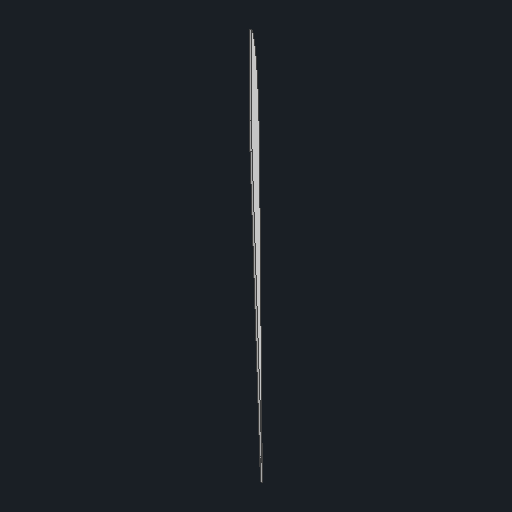
# Autodesk Inventor part: standoff
Saved by Autodesk Inventor 2023 (Build 270158030, 158C)
## iProperties
Created: 2022-03-24
Part Number: standoff
Material: Generic
Document SubType Name: Modeling
Designer: kardo
Density: 1 g/cm^3
Appearance: Default
Author: kardo
Autodesk Inventor part; units mm, degrees
ref_plane "YZ Plane" through (0, 0, 0) normal (1, 0, 0) x (0, 1, 0)
ref_plane "XZ Plane" through (0, 0, 0) normal (0, 1, 0) x (-1, 0, 0)
ref_plane "XY Plane" through (0, 0, 0) normal (0, 0, 1) x (1, 0, 0)
derived "parameters_frame.ipt"
derived "surface_body.ipt"
sketch "sk_rail_bottom_standoff" plane through (34.32, 0, 0) normal (1, 0, 0) x (0, 1, 0)
  line L0 (-345, 16.32) -> (-262.2001, 18.586)
  arc A0 (-262.2001, 18.586) -> (-241.5001, 19.2432) centre (-326.8578, 2381.2399) ccw
  line L1 (36.465, 28.832) -> (112.2, 28.832)
  arc A1 (36.465, 28.832) -> (11.22, 28.376) centre (36.465, -670.197) ccw
  line L2 (-241.5001, 19.2432) -> (11.22, 28.376)
  line L3 (-465, 0) -> (375, 0) construction
  line L4 (11.22, 28.376) -> (11.22, 0) construction
  line L5 (-241.5001, 19.2432) -> (-241.5001, 0) construction
  point P0 (0, 0)
  point P1 (-241.5001, 19.1524)
  point P2 (11.22, 28.832)
sketch "sk_rail_standoff_standoff" plane through (34.32, 0, 0) normal (1, 0, 0) x (0, 1, 0)
  line L0 (0, 21.3303) -> (92.004, 22.2293) construction
  line L1 (92.004, 22.2293) -> (112.2, 28.832) construction
  line L2 (0, 21.3303) -> (-241.5001, 18.9703)
  line L3 (-262.2001, 18.586) -> (-345, 16.32)
  arc A0 (-241.5001, 18.9703) -> (-262.2001, 18.586) centre (-229.9974, -1158.1286) ccw
  line L4 (-465, 0) -> (375, 0) construction
  line L5 (-241.5001, 18.9703) -> (-241.5001, 0) construction
  spline S0 degree 2 poles (0, 21.3303) (92.004, 22.2293) (112.2, 28.832) knots 1 1 1 2 2 2
  point P0 (0, 0)
  point P1 (-241.5001, 19.1524)
ref_plane "plane_standoff_right" through (34.32, 0, 0) normal (1, 0, 0) x (0, 1, 0)
sketch "sk_base" plane through (34.32, 0, 0) normal (1, 0, 0) x (0, 1, 0)
  arc A0 (-241.5001, 18.9703) -> (-262.2001, 18.586) centre (-229.9974, -1158.1286) ccw construction
  arc A1 (-262.2001, 18.586) -> (-241.5001, 19.2432) centre (-326.8578, 2381.2399) ccw construction
  line L0 (-241.5001, 19.2432) -> (11.22, 28.376) construction
  line L1 (0, 21.3303) -> (-241.5001, 18.9703) construction
  spline S0 degree 2 poles (0, 21.3303) (92.004, 22.2293) (112.2, 28.832) knots 1 1 1 2 2 2 construction
  line L2 (36.465, 28.832) -> (112.2, 28.832) construction
  arc A2 (36.465, 28.832) -> (11.22, 28.376) centre (36.465, -670.197) ccw construction
  line L3 (-0.0117, 22.5302) -> (-241.5118, 20.1702)
  arc A3 (-241.5118, 20.1702) -> (-262.2001, 19.7864) centre (-229.9974, -1158.1286) ccw
  arc A4 (-262.2001, 19.7864) -> (-241.5434, 20.4424) centre (-326.8578, 2381.2399) ccw
  line L4 (-241.5434, 20.4424) -> (11.1767, 29.5752)
  arc A5 (36.465, 30.032) -> (11.1767, 29.5752) centre (36.465, -670.197) ccw
  line L5 (36.465, 30.032) -> (110.2, 30.032)
  line L6 (-262.2001, 18.586) -> (-262.2001, 19.7864) construction
  line L7 (110.2, 29.4835) -> (110.2, 30.032)
  spline S1 degree 5 poles (110.2, 29.4835) (108.4013, 28.9839) (106.5765, 28.5781) (104.7453, 28.2164) (99.6086, 27.3208) (94.4369, 26.6545) (91.1112, 26.2813) (83.3135, 25.5106) (75.499, 24.9302) (71.019, 24.6404) (60.9107, 24.0665) (50.795, 23.6408) (45.1633, 23.4386) (32.751, 23.0574) (20.3354, 22.7975) (13.5533, 22.6845) (6.7709, 22.5965) (-0.0117, 22.5302) knots 0 0 0 0 0 0 0.084396 0.084396 0.084396 0.235664 0.235664 0.235664 0.438609 0.438609 0.438609 0.69336 0.69336 0.69336 1 1 1 1 1 1
  point P0 (0, 0)
  dimension "d5" = 1.2
  dimension "d4" = 1.2
  dimension "d6" = 2
  constraints: 10 end point, 6 point on circle, 3 centre point, 2 vertical, 1 parallel, 7 other
  measures "d4" distance between parallel lines of L0 L4
  measures "d6" distance from line of L7 point (112.2, 28.832)
extrude "thicken" add sketch "sk_base" against normal blind 2
equation "\"d4\" = shell_thickness"
equation "\"d6\" = bulkhead_thickness"
equation "\"d2\" = bulkhead_thickness"
equation "\"shell_thickness\" = 1.2"
equation "\"bulkhead_thickness\" = 2"
body "Solid1"
